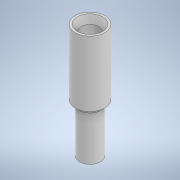
# Autodesk Inventor part: ENDER 3 HEATBREAK
Saved by Autodesk Inventor 2022 (Build 260153070, 153G)
## iProperties
Created: 2022-01-01
Part Number: ENDER 3 HEATBREAK
Material: Generic
Document SubType Name: Modeling
Designer: a laptop
Density: 1 g/cm^3
Appearance: Default
Author: a laptop
Autodesk Inventor part; units mm, degrees
ref_plane "YZ Plane" through (0, 0, 0) normal (1, 0, 0) x (0, 1, 0)
ref_plane "XZ Plane" through (0, 0, 0) normal (0, 1, 0) x (-1, 0, 0)
ref_plane "XY Plane" through (0, 0, 0) normal (0, 0, 1) x (1, 0, 0)
sketch "Sketch1" plane through (0, 0, 0) normal (0, 0, 1) x (1, 0, 0)
  line L0 (-3.5, 27) -> (-3.5, 11.55)
  line L1 (-3.5, 11.55) -> (-2.45, 10.5)
  line L2 (-2.45, 10.5) -> (-2.45, 0)
  line L3 (-2.45, 0) -> (0, 0)
  line L4 (0, 27) -> (0, 0) construction
  line L5 (-3, 27) -> (-2.1, 25.4412)
  line L6 (-2.1, 25.4412) -> (-2.1, 0)
  line L7 (-3, 27) -> (-3.5, 27)
  dimension "d1" = 10.5
  dimension "d2" = 2.45
  dimension "d3" = 3.5
  dimension "d4" = 30
  dimension "d5" = 2.1
  dimension "d6" = 135
  dimension "d7" = 0.5
  dimension "d8" = 27
  constraints: 16 end point, 3 perpendicular, 2 horizontal alignment, 2 parallel, 1 coincident, 1 horizontal, 1 point on line
  measures "d1" distance of L1.end L2.end
  measures "d2" distance of L2.end L3.end
  measures "d3" distance of L4.start L0.start
  measures "d4" angle of L4 L5
  measures "d5" distance between parallel lines of L4 L6
  measures "d6" angle of L0 L1
  measures "d7" distance of L5.start L0.start
  measures "d8" vertical distance of L2.end L0.start
revolve "Revolution1" add sketch "Sketch1" angle 360 about axis through (0, 27, 0) along (0, -1, 0)
body "Solid1"
